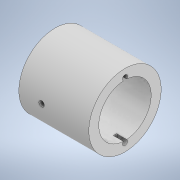
# Autodesk Inventor part: porca redonda
Saved by Autodesk Inventor 2022.1 (Build 261234020, 234B)
## iProperties
Created: 2023-08-18
Part Number: porca redonda
Material: Generic
Document SubType Name: Modeling
Designer: SENAI
Density: 1 g/cm^3
Appearance: Default
Author: SENAI
Autodesk Inventor part; units mm, degrees
ref_plane "YZ Plane" through (0, 0, 0) normal (1, 0, 0) x (0, 1, 0)
ref_plane "XZ Plane" through (0, 0, 0) normal (0, 1, 0) x (-1, 0, 0)
ref_plane "XY Plane" through (0, 0, 0) normal (0, 0, 1) x (1, 0, 0)
sketch "Sketch1" plane through (0, 0, 0) normal (0, 0, 1) x (1, 0, 0)
  line L0 (0, 0) -> (87, 0)
  line L1 (0, 0) -> (0, 45)
  line L2 (0, 45) -> (87, 45)
  line L3 (87, 45) -> (87, 0)
  dimension "d0" = 87
  dimension "d2" = 45
  constraints: 8 end point, 2 perpendicular, 1 horizontal, 1 vertical
  measures "d0" distance of L0.start L0.end
  measures "d2" distance of L0.start L1.end
revolve "Revolution1" add sketch "Sketch1" angle 360 about axis through (0, 0, 0) along (1, 0, 0)
sketch "Sketch2" plane through (87, 0, 0) normal (1, 0, 0) x (0, 0, -1)
  circle A0 centre (0, 0) radius 32.6
  dimension "d4" = 65.2
  constraints: 1 centre point, 1 coincident
  measures "d4" diameter of A0
extrude "Extrusion1" cut sketch "Sketch2" against normal through all
sketch "Sketch3" plane through (0, 0, 0) normal (-1, 0, 0) x (0, 0, 1)
  point P0 (0, 0)
sketch "Sketch4" plane through (0, 0, 0) normal (-1, 0, 0) x (0, 0, 1)
  circle A0 centre (0, 0) radius 40
  dimension "d7" = 80
  constraints: 1 centre point, 1 coincident
  measures "d7" diameter of A0
extrude "Extrusion2" cut sketch "Sketch4" against normal blind 15.5
sketch "Sketch5" plane through (87, 0, 0) normal (1, 0, 0) x (0, 0, -1)
  circle A0 centre (0, 35) radius 3.2
  circle A1 centre (0, -35) radius 3.2
  point P0 (0, 0)
  dimension "d12" = 6.4
  dimension "d13" = 6.4
  constraints: 2 centre point
  measures "d12" diameter of A0
  measures "d13" diameter of A1
extrude "Extrusion3" cut sketch "Sketch5" against normal blind 12.4
sketch "Sketch6" plane through (0, 0, 0) normal (0, 0, 1) x (1, 0, 0)
  circle A0 centre (28.3, 0) radius 3.4
  point P0 (0, 0)
  dimension "d17" = 6.8
  constraints: 1 centre point
  measures "d17" diameter of A0
extrude "Extrusion4" cut sketch "Sketch6" along normal through all
body "Solid1"
